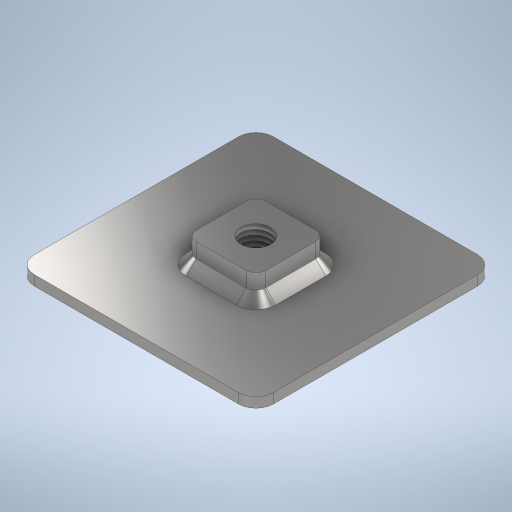
# Autodesk Inventor part: Bottom_contact
Saved by Autodesk Inventor 2023 (Build 270158000, 158)
## iProperties
Created: 2022-09-20
Part Number: Bottom_contact
Material: Сталь нержавеющая AISI 202
Document SubType Name: Modeling
Designer: Makar
Density: 7.85472 g/cm^3
Appearance: С умеренной полировкой
Author: Makar
Autodesk Inventor part; units mm, degrees
ref_plane "YZ Plane" through (0, 0, 0) normal (1, 0, 0) x (0, 1, 0)
ref_plane "XZ Plane" through (0, 0, 0) normal (0, 1, 0) x (-1, 0, 0)
ref_plane "XY Plane" through (0, 0, 0) normal (0, 0, 1) x (1, 0, 0)
sketch "Эскиз1" plane through (0, 0, 0) normal (0, 1, 0) x (-1, 0, 0)
  line L0 (4.5, 0) -> (45.5, 0)
  line L1 (50, 4.5) -> (50, 45.5)
  line L2 (45.5, 50) -> (4.5, 50)
  line L3 (0, 45.5) -> (0, 4.5)
  arc A0 (50, 45.5) -> (45.5, 50) centre (45.5, 45.5) ccw
  arc A1 (45.5, 0) -> (50, 4.5) centre (45.5, 4.5) ccw
  arc A2 (4.5, 50) -> (0, 45.5) centre (4.5, 45.5) ccw
  arc A3 (0, 4.5) -> (4.5, 0) centre (4.5, 4.5) ccw
  point P0 (0, 0)
  point P1 (50, 50)
  point P2 (50, 0)
  point P3 (0, 50)
  dimension "d0" = 50
  dimension "d1" = 50
  dimension "d2" = 4.5
  dimension "d3" = 4.5
  dimension "d4" = 4.5
  dimension "d5" = 4.5
  constraints: 8 end point, 8 point on circle, 8 point on line, 8 tangent, 4 centre point, 2 parallel, 1 horizontal, 1 perpendicular
  measures "d0" distance of point (0, 50) point (50, 50)
  measures "d1" distance of point (50, 50) point (50, 0)
  measures "d2" radius of A0
  measures "d3" radius of A1
  measures "d4" radius of A2
  measures "d5" radius of A3
extrude "Выдавливание1" add sketch "Эскиз1" along normal blind 2
sketch "Эскиз2" plane through (0, 2, 0) normal (0, 1, 0) x (1, 0, 0)
  line L0 (-50, -4.5) -> (-50, -45.5) projected
  line L1 (-50, -25) -> (0, -25)
  line L2 (0, -45.5) -> (0, -4.5) projected
  circle A0 centre (-25, -25) radius 3
  arc A1 (-45.5, 0) -> (-50, -4.5) centre (-45.5, -4.5) ccw projected
  line L3 (-50, -4.5) -> (-50, -45.5) projected
  arc A2 (-50, -45.5) -> (-45.5, -50) centre (-45.5, -45.5) ccw projected
  line L4 (-45.5, -50) -> (-4.5, -50) projected
  arc A3 (-4.5, -50) -> (0, -45.5) centre (-4.5, -45.5) ccw projected
  line L5 (0, -45.5) -> (0, -4.5) projected
  arc A4 (0, -4.5) -> (-4.5, 0) centre (-4.5, -4.5) ccw projected
  line L6 (-4.5, 0) -> (-45.5, 0) projected
  line L7 (-30, -32) -> (-20, -32)
  line L8 (-18, -30) -> (-18, -20)
  line L9 (-20, -18) -> (-30, -18)
  line L10 (-32, -20) -> (-32, -30)
  line L11 (-32, -32) -> (-18, -18) construction
  line L12 (-18, -32) -> (-32, -18) construction
  arc A5 (-30, -18) -> (-32, -20) centre (-30, -20) ccw
  arc A6 (-32, -30) -> (-30, -32) centre (-30, -30) ccw
  arc A7 (-20, -32) -> (-18, -30) centre (-20, -30) ccw
  arc A8 (-18, -20) -> (-20, -18) centre (-20, -20) ccw
  point P0 (0, 0)
  dimension "d8" = 6
  dimension "d9" = 14
  dimension "d10" = 14
  dimension "d11" = 2
  dimension "d12" = 2
  constraints: 14 end point, 8 point on circle, 8 point on line, 8 tangent, 5 centre point, 5 midpoint, 2 equal radius, 2 parallel, 1 horizontal, 1 perpendicular
  measures "d8" diameter of A0
  measures "d9" distance of L12.end L11.end
  measures "d10" distance of L11.end L12.start
  measures "d11" radius of A5
  measures "d12" radius of A6
extrude "Выдавливание2" add sketch "Эскиз2" along normal blind 5 contours L10 A5 L9 A8 L8 L1 A0 | L1 A0 L8 A7 L7 A6 L10
chamfer "Фаска1" distance 2 angle 45 8 edges at (-25, 2, 32) (-31.4142, 2, 31.4142) (-32, 2, 25) (-31.4142, 2, 18.5858) (-25, 2, 18) (-18.5858, 2, 18.5858) (-18, 2, 25) (-18.5858, 2, 31.4142)
extrude "Выдавливание3" cut sketch "Эскиз2" against normal blind 5 contours A0 L1 | L1 A0
thread "Резьба1" size "M6x1" class "6H" standard "ANSI Metric M Profile" full length
sketch "Эскиз3" plane through (0, 2, 0) normal (0, 1, 0) x (1, 0, 0)
  arc A0 (-45.5, 0) -> (-50, -4.5) centre (-45.5, -4.5) ccw projected
  line L0 (-50, -4.5) -> (-50, -45.5) projected
  arc A1 (-50, -45.5) -> (-45.5, -50) centre (-45.5, -45.5) ccw projected
  line L1 (-45.5, -50) -> (-4.5, -50) projected
  arc A2 (-4.5, -50) -> (0, -45.5) centre (-4.5, -45.5) ccw projected
  line L2 (0, -45.5) -> (0, -4.5) projected
  arc A3 (0, -4.5) -> (-4.5, 0) centre (-4.5, -4.5) ccw projected
  line L3 (-4.5, 0) -> (-45.5, 0) projected
  line L4 (-30, -34) -> (-20, -34) projected
  arc A4 (-34, -30) -> (-30, -34) centre (-30, -30) ccw projected
  line L5 (-34, -20) -> (-34, -30) projected
  arc A5 (-30, -16) -> (-34, -20) centre (-30, -20) ccw projected
  line L6 (-20, -16) -> (-30, -16) projected
  arc A6 (-16, -20) -> (-20, -16) centre (-20, -20) ccw projected
  line L7 (-16, -30) -> (-16, -20) projected
  arc A7 (-20, -34) -> (-16, -30) centre (-20, -30) ccw projected
  line L8 (-1, -4.5) -> (-1, -45.5)
  arc A8 (-4.5, -49) -> (-1, -45.5) centre (-4.5, -45.5) ccw
  line L9 (-4.5, -49) -> (-45.5, -49)
  arc A9 (-49, -45.5) -> (-45.5, -49) centre (-45.5, -45.5) ccw
  line L10 (-49, -45.5) -> (-49, -4.5)
  arc A10 (-45.5, -1) -> (-49, -4.5) centre (-45.5, -4.5) ccw
  line L11 (-45.5, -1) -> (-4.5, -1)
  arc A11 (-1, -4.5) -> (-4.5, -1) centre (-4.5, -4.5) ccw
  point P0 (0, 0)
  dimension "d22" = 1
  constraints: 8 end point, 8 point on circle, 4 centre point, 7 other
  measures "d22" distance between parallel lines of L2 L8
extrude "Выдавливание4" cut sketch "Эскиз3" against normal blind 10 contours L3 A3 L2 A2 L1 A1 L0 A0
